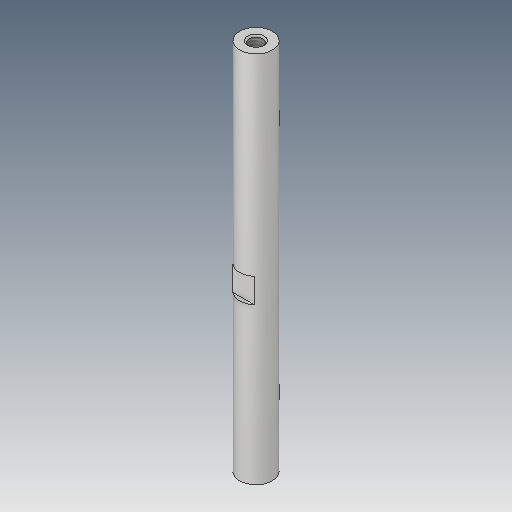
# Autodesk Inventor part: p8ALshaftP
Saved by Autodesk Inventor 2019.4 (Build 234330000, 330)
## iProperties
Created: 2019-06-11
Part Number: p8ALshaftP
Material: アルミニウム 2014-T4
Document SubType Name: Modeling
Designer: AzLIer
Density: 2.8 g/cm^3
Appearance: サテン
Mass: 12.0151 g
Surface Area: 26.8707 cm^2
Volume: 4.29111 cm^3
Author: AzLIer
Autodesk Inventor part; units mm, degrees
ref_plane "YZ Plane" through (0, 0, 0) normal (1, 0, 0) x (0, 1, 0)
ref_plane "XZ Plane" through (0, 0, 0) normal (0, 1, 0) x (-1, 0, 0)
ref_plane "XY Plane" through (0, 0, 0) normal (0, 0, 1) x (1, 0, 0)
sketch "スケッチ1" plane through (0, 0, 0) normal (0, 1, 0) x (-1, 0, 0)
  circle A0 centre (0, 0) radius 4
  dimension "d0" = 8
  constraints: 1 centre point, 1 coincident
  measures "d0" diameter of A0
extrude "押し出し1" add sketch "スケッチ1" along normal blind 91
sketch "スケッチ2" plane through (0, 0, 0) normal (0, -1, 0) x (1, 0, 0)
  point P0 (0, 0)
sketch "スケッチ3" plane through (0, 91, 0) normal (0, 1, 0) x (1, 0, 0)
  point P0 (0, 0)
hole "穴1" at (0, 91, 0) direction (0, -1, 0) diameter 3.242 depth 14 tip angle 118 countersink diameter 4 countersink angle 90 thread size "M4x0.7" class "6H" standard "ISO Metric profile"
hole "穴2" at (0, 0, 0) direction (0, 1, 0) diameter 3.242 depth 14 tip angle 118 countersink diameter 4 countersink angle 90 thread size "M4x0.7" class "6H" standard "ISO Metric profile"
sketch "スケッチ4" plane through (0, 0, 0) normal (1, 0, 0) x (0, 1, 0)
  line L0 (76, -4) -> (76, 4) projected
  spline S0 degree 3 poles (39, 7.4285) (39, 7.3385) (39.0585, 7.233) (39.2835, 7.0254) (39.4498, 6.9237) (39.8139, 6.7628) (40.035, 6.6916) (40.51, 6.5961) (40.7638, 6.5723) (41.2362, 6.5723) (41.49, 6.5961) (41.965, 6.6916) (42.1861, 6.7628) (42.5502, 6.9237) (42.7165, 7.0254) (42.9415, 7.233) (43, 7.3385) (43, 7.4285) knots 0.287107 0.287107 0.287107 0.287107 0.359812 0.359812 0.432516 0.432516 0.503365 0.503365 0.574214 0.574214 0.645063 0.645063 0.715911 0.715911 0.788616 0.788616 0.861321 0.861321 0.861321 0.861321 projected
  line L1 (15, 4) -> (15, -4) projected
  line L2 (76, -3) -> (72.8, -3)
  line L3 (72.8, -3) -> (72.8, -4)
  line L4 (72.8, -4) -> (76, -4)
  line L5 (44, 4) -> (38, 4)
  line L6 (38, 4) -> (38, 3)
  line L7 (38, 3) -> (44, 3)
  line L8 (44, 3) -> (44, 4)
  line L9 (43, 7.4285) -> (39, 7.4285)
  line L10 (15, -4) -> (18.2, -4)
  line L11 (18.2, -4) -> (18.2, -3)
  line L12 (18.2, -3) -> (15, -3)
  line L13 (15, -3) -> (15, -4)
  point P0 (0, 0)
  point P1 (41, 7.4285)
  point P2 (41, 4)
  dimension "d17" = 3.2
  dimension "d18" = 1
  dimension "d19" = 6
  constraints: 24 end point, 5 perpendicular, 4 parallel, 3 equal length, 3 horizontal, 2 midpoint, 2 point on line, 1 vertical alignment
  measures "d17" distance of L3.end L0.start
  measures "d18" distance of L2.end L3.end
  measures "d19" distance of L6.end L7.end
extrude "押し出し2" cut sketch "スケッチ4" along normal through all both and the other way through all contours L4 L3 L2 L0 | L12 L11 L10 L1 | L8 L7 L6 L5
